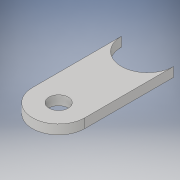
# Autodesk Inventor part: chain_elmt_1
Saved by Autodesk Inventor 2019.3 (Build 233278000, 278)
## iProperties
Created: 2020-08-28
Part Number: chain_elmt_1
Material: Generisch
Document SubType Name: Modeling
Designer: Nicolas Frick
Density: 1 g/cm^3
Appearance: Vorgabe
Author: Nicolas Frick
Autodesk Inventor part; units mm, degrees
ref_plane "YZ Plane" through (0, 0, 0) normal (1, 0, 0) x (0, 1, 0)
ref_plane "XZ Plane" through (0, 0, 0) normal (0, 1, 0) x (-1, 0, 0)
ref_plane "XY Plane" through (0, 0, 0) normal (0, 0, 1) x (1, 0, 0)
sketch "Skizze1" plane through (0, 0, 0) normal (0, 1, 0) x (-1, 0, 0)
  circle A0 centre (0, 0) radius 1.85
  circle A1 centre (0, 0) radius 5
  line L0 (0, 0) -> (0, -12) construction
  arc A2 (5, -17) -> (-5, -17) centre (0, -17) ccw
  line L1 (5, 0) -> (5, -17)
  line L2 (-5, 0) -> (-5, -17)
  dimension "d0" = 3.7
  dimension "d1" = 10
  constraints: 6 end point, 5 point on circle, 3 centre point, 2 coincident, 1 parallel, 1 tangent, 1 vertical
  measures "d0" diameter of A0
  measures "d1" diameter of A1
extrude "Extrusion1" add sketch "Skizze1" along normal blind 1.8
